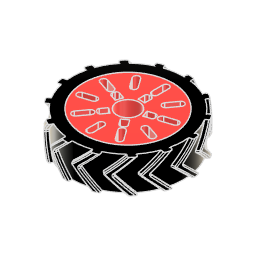
Tire (Autodesk Fusion 360 design; units mm, degrees)
Autodesk Fusion 360 part; units mm, degrees
note: some values were not read from the file. Chosen so that the rebuilt part matches the saved one: where a step starts.
sketch "Sketch1" plane through (0, 0, 0) normal (0, 0, 1) x (1, 0, 0)
  circle A0 centre (0, 0) radius 50
  circle A1 centre (0, 0) radius 40
  dimension "d1" = 100
  dimension "d2" = -10
  constraint coincident A0.centre A1.centre
  measures "d1" diameter of A0
extrude "Extrude1" add sketch "Sketch1" along normal blind 30 makes body 1
sketch "Sketch2" plane through (0, 0, 0) normal (0, 1, 0) x (1, 0, 0)
  line L0 (-50, 0) -> (50, 0)
  line L1 (-50, -30) -> (50, -30)
  line L2 (0, 0) -> (0, -30) construction
  line L3 (0, -15) -> (-15, -15) construction
  line L4 (-15, -15) -> (0, 0)
  line L5 (0, -30) -> (-15, -15)
  line L6 (-6.364, -30) -> (-21.364, -15)
  line L7 (-21.364, -15) -> (-6.364, 0)
  dimension "d5" = 15
  constraint coincident L2.start L4.end
  constraint midpoint L1 L2.end
  constraint midpoint L2 L3.start
  constraint perpendicular L2 L3
  constraint coincident L0 L7.end
  constraint coincident L1 L6.start
  measures "d5" distance of L3.start L3.end
extrude "Extrude2" add sketch "Sketch2" against normal blind 3.5 from the far side of the face at (49.7515, -4.9784, 20) on bodies 1 bodies 1
fillet "Fillet1" radius 1 6 edges at (-21.364, -46.956, 15) (-14.0364, -51.4894, 22.3275) (-7.5879, -52.9209, 7.5879) (-14.0364, -51.4894, 7.6725) (-7.5879, -52.9209, 22.4121) (-15, -49.447, 15) on bodies 1
pattern_circular "C-Pattern1" count 14 over 360 about axis through (0, 0, 1.75) along (0, 0, 1) of "Extrude2", "Fillet1"
extrude "Extrude3" add sketch "Sketch1" along normal blind 30 separate body contours A1 makes body 2
sketch "Sketch3" plane through (0, 0, 30) normal (0, 0, 1) x (-1, 0, 0)
  circle A0 centre (0, 0) radius 40
  circle A1 centre (0, 0) radius 10
  dimension "d15" = 20
  constraint coincident A0.centre A1.centre
  measures "d15" diameter of A1
extrude "Extrude4" cut sketch "Sketch3" against normal through all contours A1 bodies 2
sketch "Sketch4" plane through (0, 0, 30) normal (0, 0, 1) x (-1, 0, 0)
  circle A0 centre (0, 0) radius 10
  circle A1 centre (0, 0) radius 40
  circle A2 centre (0, 0) radius 40
  line L0 (0, -40) -> (0, 0)
  circle A3 centre (0, 0) radius 10
  line L1 (-3, -12) -> (3, -12)
  line L2 (3, -12) -> (3, -18)
  line L3 (1, -20) -> (-1, -20)
  line L4 (-3, -18) -> (-3, -12)
  line L5 (-3, -12) -> (3, -20) construction
  line L6 (3, -12) -> (-3, -20) construction
  arc A4 (1, -20) -> (3, -18) centre (1, -18) ccw
  arc A5 (-3, -18) -> (-1, -20) centre (-1, -18) ccw
  point P0 (0, -16)
  dimension "d17" = 6
  dimension "d18" = 8
  dimension "d19" = 2
  constraint coincident A0.centre A1.centre
  constraint coincident A2 L0.start
  constraint vertical L0
  constraint horizontal L1
  constraint perpendicular L1 L2
  constraint parallel L1 L3
  constraint parallel L2 L4
  constraint coincident L5 P0
  constraint coincident L6 P0
  constraint coincident L0 P0
  constraint coincident L5.end L2
  constraint coincident L5.end L3
  constraint tangent L2 A4
  constraint tangent L3 A4
  constraint coincident L6.end L4
  constraint coincident L6.end L3
  constraint tangent L4 A5
  constraint tangent L3 A5
  constraint equal A4 A5
  measures "d17" distance of L5.end L6.end
  measures "d18" distance of L1.end L5.end
  measures "d19" radius of A4
extrude "Extrude5" cut sketch "Sketch4" against normal through all contours L0 L1 L3 L4 A5 | L0 L1 L2 L3 A4 bodies 2
pattern_circular "C-Pattern2" count 5 over 360 about axis through (0, 0, 1.75) along (0, 0, 1) of "Extrude5"
sketch "Sketch5" plane through (0, 0, 30) normal (0, 0, 1) x (-1, 0, 0)
  line L0 (-10.4856, -6.5614) -> (-16.192, -8.4155)
  arc A0 (-18.7121, -7.1314) -> (-16.192, -8.4155) centre (-16.81, -6.5134) ccw
  line L1 (-18.7121, -7.1314) -> (-19.3301, -5.2293)
  arc A1 (-18.0461, -2.7091) -> (-19.3301, -5.2293) centre (-17.428, -4.6112) ccw
  line L2 (-18.0461, -2.7091) -> (-12.3397, -0.855)
  line L3 (-12.3397, -0.855) -> (-10.4856, -6.5614)
  line L4 (-9.4805, 7.9448) -> (-13.0072, 12.799)
  arc A2 (-12.5647, 15.5926) -> (-13.0072, 12.799) centre (-11.3892, 13.9745) ccw
  line L5 (-12.5647, 15.5926) -> (-10.9467, 16.7681)
  arc A3 (-8.1531, 16.3257) -> (-10.9467, 16.7681) centre (-9.7711, 15.1501) ccw
  line L6 (-8.1531, 16.3257) -> (-4.6264, 11.4716)
  line L7 (-4.6264, 11.4716) -> (-9.4805, 7.9448)
  line L8 (4.6264, 11.4716) -> (8.1531, 16.3257)
  arc A4 (10.9467, 16.7681) -> (8.1531, 16.3257) centre (9.7711, 15.1501) ccw
  line L9 (10.9467, 16.7681) -> (12.5647, 15.5926)
  arc A5 (13.0072, 12.799) -> (12.5647, 15.5926) centre (11.3892, 13.9745) ccw
  line L10 (13.0072, 12.799) -> (9.4805, 7.9448)
  line L11 (9.4805, 7.9448) -> (4.6264, 11.4716)
  line L12 (12.3397, -0.855) -> (18.0461, -2.7091)
  arc A6 (19.3301, -5.2293) -> (18.0461, -2.7091) centre (17.428, -4.6112) ccw
  line L13 (19.3301, -5.2293) -> (18.7121, -7.1314)
  arc A7 (16.192, -8.4155) -> (18.7121, -7.1314) centre (16.81, -6.5134) ccw
  line L14 (16.192, -8.4155) -> (10.4856, -6.5614)
  line L15 (10.4856, -6.5614) -> (12.3397, -0.855)
  line L16 (3, -12) -> (3, -18)
  arc A8 (1, -20) -> (3, -18) centre (1, -18) ccw
  line L17 (1, -20) -> (-1, -20)
  arc A9 (-3, -18) -> (-1, -20) centre (-1, -18) ccw
  line L18 (-3, -18) -> (-3, -12)
  line L19 (-3, -12) -> (3, -12)
  circle A10 centre (0, 0) radius 10
  circle A11 centre (0, 0) radius 40
  line L20 (-2.75, -24) -> (-2.75, -34)
  arc A12 (-2.75, -34) -> (2.75, -34) centre (0, -34) ccw
  line L21 (2.75, -34) -> (2.75, -24)
  arc A13 (2.75, -24) -> (-2.75, -24) centre (0, -24) ccw
  line L22 (0, -24) -> (0, -34) construction
  dimension "d23" = 5.5
  constraint tangent L20 A12
  constraint tangent A12 L21
  constraint parallel L20 L21
  constraint tangent L21 A13
  constraint tangent L20 A13
  constraint vertical L22
  measures "d23" diameter of A12
extrude "Extrude6" cut sketch "Sketch5" against normal through all contours L20 A12 L21 A13 bodies 2
pattern_circular "C-Pattern3" count 10 over 360 about axis through (0, 0, 1.75) along (0, 0, 1) of "Extrude6"
